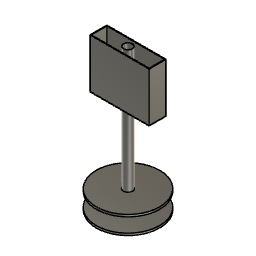
Cuerpo v1 (Autodesk Fusion 360 design; units mm, degrees)
Autodesk Fusion 360 part; units mm, degrees
sketch "Boceto1" plane through (0, 0, 0) normal (0, 1, 0) x (1, 0, 0)
  line L0 (0, 0) -> (0, -1000)
  line L1 (0, 0) -> (32.5, 0)
  line L2 (32.5, -1000) -> (0, -1000)
  line L3 (0, 0) -> (225, 0)
  line L4 (225, 0) -> (225, -15)
  line L5 (225, -15) -> (32.5, -15)
  line L6 (32.5, -115) -> (225, -115)
  line L7 (225, -115) -> (225, -130)
  line L8 (225, -130) -> (32.5, -130)
  line L9 (32.5, -650) -> (210, -650)
  line L10 (32.5, -15) -> (32.5, -115)
  line L11 (32.5, -130) -> (32.5, -1000)
  dimension "d1" = 1000
  dimension "d2" = 32.5
  dimension "d3" = 225
  dimension "d4" = 15
  dimension "d5" = 15
  dimension "d6" = 192.5
  dimension "d7" = 100
  dimension "d9" = 650
  constraint coincident L0.start L1.start
  constraint vertical L0
  constraint perpendicular L0 L1
  constraint perpendicular L1 L10
  constraint perpendicular L0 L2
  constraint perpendicular L0 L3
  constraint perpendicular L3 L4
  constraint perpendicular L5 L10
  constraint perpendicular L6 L10
  constraint perpendicular L6 L7
  constraint coincident L8.end L10
  constraint perpendicular L8 L10
  constraint perpendicular L0 L9
  constraint coincident L9.start L10
  constraint collinear L10 L11
  measures "d1" distance of L0.start L0.end
  measures "d2" distance of L0.start L1.end
  measures "d3" distance of L0.start L3.end
  measures "d4" distance of L3.end L4.end
  measures "d5" distance of L6.end L7.end
  measures "d6" distance of L7.end L8.end
  measures "d7" distance of L5 L6
  measures "d9" distance of L3 L9
revolve "Revolución1" add sketch "Boceto1" angle 360 about axis through (0, 0, 0) along (0, 0, 1)
extrude "Extruir1" cut 1 faces at (-1.1612, 8.4698, 1000) along direction (0, 0, -1) blind 350
sketch "Boceto2" plane through (0, 0, 650) normal (0, 0, 1) x (-1, 0, 0)
  circle A0 centre (0, 0) radius 32.5
  line L0 (210, 0) -> (210, -60)
  line L1 (210, -60) -> (-210, -60)
  line L2 (-210, -60) -> (-210, 60)
  line L3 (-210, 60) -> (210, 60)
  line L4 (210, 60) -> (210, 0)
  dimension "d13" = 210
  dimension "d14" = 60
  dimension "d15" = 420
  dimension "d16" = 120
  dimension "d17" = 420
  constraint perpendicular L0 L1
  constraint perpendicular L1 L2
  constraint perpendicular L2 L3
  measures "d13" distance of A0.centre L0.start
  measures "d14" distance of L0.start L0.end
  measures "d15" distance of L0.end L1.end
  measures "d16" distance of L1.end L2.end
  measures "d17" distance of L2.end L3.end
extrude "Extruir2" add sketch "Boceto2" 1 faces at (-1.1612, 8.4698, 650) along normal blind 350
sketch "Boceto3" plane through (0, 0, 1000) normal (0, 0, 1) x (-1, 0, 0)
  line L0 (210, 60) -> (-210, 60)
  line L1 (-210, 60) -> (-210, -60)
  line L2 (-210, -60) -> (210, -60)
  line L3 (210, -60) -> (210, 60)
  circle A0 centre (0, 0) radius 32.5
  dimension "d20" = 65
  constraint coincident A0.centre origin
  measures "d20" diameter of A0
sketch "Boceto4" plane through (0, 0, 1000) normal (0, 0, 1) x (-1, 0, 0)
  circle A0 centre (0, 0) radius 30
  dimension "d21" = 60
  constraint coincident A0.centre origin
  measures "d21" diameter of A0
extrude "Extruir3" cut sketch "Boceto4" against normal blind 1000
sketch "Boceto5" plane through (0, 0, 0) normal (0, 0, -1) x (1, 0, 0)
  circle A0 centre (0, 0) radius 30
  circle A1 centre (0, 0) radius 225
extrude "Extruir4" add sketch "Boceto5" against normal blind 15 contours A0
sketch "Boceto6" plane through (0, -60, 0) normal (0, -1, 0) x (1, 0, 0)
  line L0 (-210, 650) -> (210, 650)
  line L1 (210, 650) -> (210, 1000)
  line L2 (210, 1000) -> (-210, 1000)
  line L3 (-210, 1000) -> (-210, 650)
sketch "Boceto7" plane through (0, 0, 1000) normal (0, 0, 1) x (-1, 0, 0)
  line L0 (205, -55) -> (205, 55)
  line L1 (205, 55) -> (-205, 55)
  line L2 (-205, 55) -> (-205, -55)
  line L3 (-205, -55) -> (205, -55)
  line L4 (210, -60) -> (210, 60)
  line L5 (-210, 60) -> (-210, -60)
  line L6 (-210, -60) -> (210, -60)
  line L7 (210, 60) -> (-210, 60)
  dimension "d26" = 5
  dimension "d27" = 5
  dimension "d28" = 5
  dimension "d29" = 5
  constraint vertical L0
  constraint perpendicular L0 L1
  constraint perpendicular L1 L2
  constraint perpendicular L0 L3
  measures "d26" distance of L0 L4
  measures "d27" distance of L2 L5
  measures "d28" distance of L3 L6
  measures "d29" distance of L1 L7
extrude "Extruir5" cut sketch "Boceto7" against normal blind 345 contours L0 L1 L2 L3
extrude "Extruir6" cut sketch "Boceto3" against normal blind 350 thin wall 1 on the right open curves A0
sketch "Boceto10" plane through (0, 0, 0) normal (0, 1, 0) x (1, 0, 0)
  line L0 (0, 0) -> (0, -1000)
  dimension "d35" = 1000
  constraint coincident L0.start origin
  constraint vertical L0
  measures "d35" distance of L0.start L0.end
extrude "Extruir7" add 1 faces at (-30.8827, 1.5649, 655) along direction (0, 0, 1) blind 350
